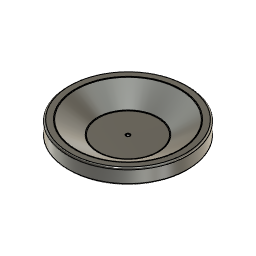
bowl disc (Autodesk Fusion 360 design; units mm, degrees)
Autodesk Fusion 360 part; units mm, degrees
sketch "Sketch1" plane through (0, 0, 0) normal (0, 1, 0) x (1, 0, 0)
  line L0 (0, 0) -> (80, -0.0047)
  line L1 (0, 0) -> (0, -2)
  line L2 (0, -2) -> (40, -2)
  line L3 (80, -0.0047) -> (79.9988, -20.0047)
  line L4 (79.9988, -20.0047) -> (69.9988, -20.0041)
  line L5 (69.9988, -20.0041) -> (40, -2)
  line L6 (0, 0) -> (2.5, 0) construction
  line L7 (2.5, 0) -> (2.5, -2)
  dimension "d3" = 2
  dimension "d5" = 20
  dimension "d6" = 10
  dimension "d10" = 2.5
  dimension "d11" = 80
  dimension "d12" = 40
  constraint perpendicular L1 L2
  constraint perpendicular L0 L3
  constraint perpendicular L3 L4
  constraint coincident L0.start L1.start
  constraint perpendicular L1 L6
  constraint coincident L2 L7.end
  constraint perpendicular L2 L7
  measures "d3" distance of L0.start L1.end
  measures "d5" distance of L0.end L3.end
  measures "d6" distance of L3.end L4.end
  measures "d10" distance of L0.start L6.end
  measures "d11" horizontal distance of L0.start L0.end
  measures "d12" distance of L1.end L2.end
revolve "Revolve1" add sketch "Sketch1" angle 360 about axis through (0, 0, 1.75) along (0, 0, 1) contours L0 L2 L3 L4 L5 L7
fillet "Fillet1" radius 2 3 faces at (43.9825, -40.8098, 14.0027) (76.5702, -3.8215, 20.0045) (79.9006, -3.9877, 6.6713)
fillet "Fillet2" radius 0.25 2 edges at (-2.3308, -0.904, 0.0001) (-2.3308, -0.904, 2)
named bodies: "Bowl Disc"
